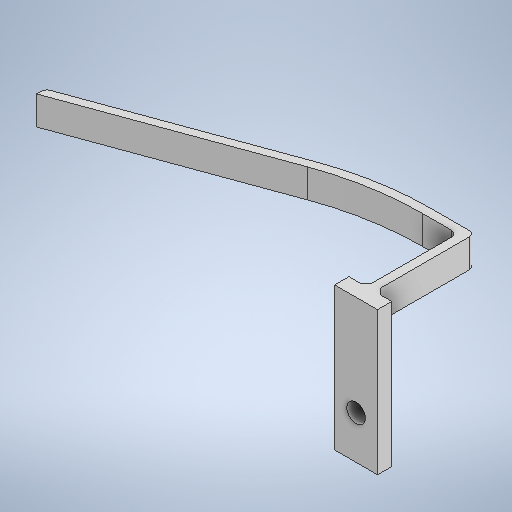
# Autodesk Inventor part: srovnavac
Saved by Autodesk Inventor 2025 (Build 290162000, 162)
## iProperties
Created: 2025-02-23
Part Number: srovnavac
Material: Všeobecné
Document SubType Name: Modeling
Designer: lukas
Density: 1 g/cm^3
Appearance: Výchozí
Author: lukas
## iProperties of the stored document srovnavac_3D tisk.ipt
Part Number: srovnavac_3D tisk
Autodesk Inventor part; units mm, degrees
ref_plane "YZ Plane" through (0, 0, 0) normal (1, 0, 0) x (0, 1, 0)
ref_plane "XZ Plane" through (0, 0, 0) normal (0, 1, 0) x (-1, 0, 0)
ref_plane "XY Plane" through (0, 0, 0) normal (0, 0, 1) x (1, 0, 0)
sketch "Náčrt1" plane through (0, 0, 0) normal (0, 0, 1) x (1, 0, 0)
  line L0 (0, 21) -> (0, -21) projected
  line L1 (-10.5, 0) -> (10.5, 0) projected
  line L2 (-7.5, 15) -> (7.5, 15)
  line L3 (7.5, 15) -> (7.5, -15)
  line L4 (7.5, -15) -> (-7.5, -15)
  line L5 (-7.5, -15) -> (-7.5, 15)
  point P0 (0, 0)
  dimension "d0" = 15
  dimension "d1" = 30
  constraints: 8 end point, 2 parallel, 1 horizontal, 1 perpendicular, 2 other
  measures "d0" distance of L2.start L2.end
  measures "d1" distance of L2.end L3.end
extrude "Vysunutí1" add sketch "Náčrt1" along normal blind 5
sketch "Náčrt2" plane through (-7.5, 15, 0) normal (0, 1, 0) x (1, 0, 0)
  line L0 (7.5, 1) -> (7.5, -6) projected
  line L1 (18, 0) -> (-3, 0) projected
  line L2 (15, 0) -> (0, 0) projected
  line L3 (0, 0) -> (0, -5) projected
  line L4 (15, -5) -> (0, -5) projected
  line L5 (15, 0) -> (15, -5) projected
  line L6 (15, 0) -> (0, 0) projected
  line L7 (0, 0) -> (15, 0)
  line L8 (15, 0) -> (15, -5)
  line L9 (15, -5) -> (0, -5)
  line L10 (0, -5) -> (0, 0)
  point P0 (7.5, 0)
  constraints: 8 end point, 2 parallel, 1 horizontal, 1 perpendicular
extrude "Vysunutí2" add sketch "Náčrt2" along normal blind 20
sketch "Náčrt3" plane through (0, 0, 5) normal (0, 0, 1) x (1, 0, 0)
  line L0 (-7.5, -15) -> (7.5, -15) projected
  line L1 (7.5, -15) -> (7.5, 35) projected
  line L2 (-7.5, 35) -> (7.5, 35) projected
  line L3 (-7.5, -15) -> (-7.5, 35) projected
  line L4 (0, 45) -> (0, -25) projected
  line L5 (-10.5, 0) -> (10.5, 0) projected
  point P0 (0, 0)
  point P1 (0, 0)
  dimension "d6" = 15
  constraints: 1 point on line
  measures "d6" distance from line of L0 point (0, 0)
hole "Díra1" at (0, 0, 5) direction (0, 0, -1) diameter 6.6 end through all
sketch "Náčrt4" plane through (-7.5, 35, 0) normal (0, 1, 0) x (1, 0, 0)
  line L0 (15, -5) -> (15, 0) projected
  line L1 (15, 0) -> (0, 0) projected
  line L2 (0, 0) -> (0, -5) projected
  line L3 (0, -5) -> (15, -5) projected
  line L4 (6, 0) -> (9, 0)
  line L5 (9, 0) -> (9, 35)
  line L6 (9, 35) -> (6, 35)
  line L7 (6, 35) -> (6, 0)
  line L8 (7.5, 43) -> (7.5, -13) projected
  line L9 (6, 35) -> (-24, 35)
  line L10 (-24, 35) -> (-24, 32)
  line L11 (-24, 32) -> (6, 32)
  line L12 (6, 32) -> (6, 35)
  line L13 (-24, 35) -> (-110, 3.6986)
  line L14 (-24, 32) -> (-110, 0.6986)
  line L15 (-110, 0.6986) -> (-110, 3.6986)
  point P0 (7.5, 0)
  point P1 (6, 32)
  dimension "d14" = 3
  dimension "d15" = 35
  dimension "d16" = 3
  dimension "d17" = 30
  dimension "d19" = 160
  dimension "d20" = 110
  constraints: 22 end point, 5 parallel, 2 horizontal, 2 perpendicular, 1 point on line, 1 vertical, 1 other
  measures "d14" distance of L5.end L6.end
  measures "d15" distance between parallel lines of L1 L6
  measures "d16" distance between parallel lines of L9 L11
  measures "d17" distance of L10.end L11.end
  measures "d19" angle of L14 L11
  measures "d20" distance between parallel lines of L2 L15
extrude "Vysunutí3" add sketch "Náčrt4" against normal blind 10 contours L1 L8 L6 L5 | L1 L7 L6 L8 | L11 L10 L9 L7 | L14 L15 L13 L10
chamfer "Zkosení1" distance 2 distance2 2 2 edges at (-1.5, 30, 0) (1.5, 30, 0) measured on face at (-6.092, 6.7993, 0)
fillet "Zaoblení2" radius 2 1 edges at (-117.5, 30, -3.6986)
fillet "Zaoblení3" radius 2 2 edges at (1.5, 30, -35) (-1.5, 30, -32)
fillet "Zaoblení4" radius 100 2 edges at (-31.5, 30, -32) (-31.5, 30, -35)
